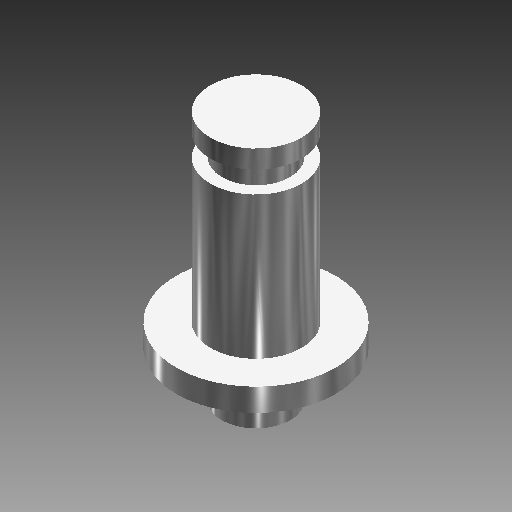
# Autodesk Inventor part: 308-16
Saved by Autodesk Inventor 2019 (Build 230136000, 136)
## iProperties
Company: Autodesk Inc.
Created: 2012-01-24
Part Number: 308-16
Material: Steel
Document SubType Name: Modeling
Designer: Autodesk Inc.
Mass: 1.16125 g
Surface Area: 2.26352 cm^2
Volume: 0.14793 cm^3
Density: 7.85 g/cm^3
Appearance: Chrome - Polished
Author: Inventor
Autodesk Inventor part; units mm, degrees
ref_plane "YZ Plane" through (0, 0, 0) normal (1, 0, 0) x (0, 1, 0)
ref_plane "XZ Plane" through (0, 0, 0) normal (0, 1, 0) x (-1, 0, 0)
ref_plane "XY Plane" through (0, 0, 0) normal (0, 0, 1) x (1, 0, 0)
sketch "Sketch1" plane through (0, 0, 0) normal (0, 0, 1) x (1, 0, 0)
  line L0 (0, 0) -> (1.5, 0)
  line L1 (1.5, 0) -> (1.5, 2)
  line L2 (1.5, 2) -> (0, 2)
  line L3 (0, 2) -> (0, 0)
  line L4 (0, 2) -> (3.5, 2)
  line L5 (3.5, 2) -> (3.5, 3)
  line L6 (3.5, 3) -> (0, 3)
  line L7 (0, 3) -> (0, 2)
  line L8 (0, 3) -> (2, 3)
  line L9 (2, 3) -> (2, 9.25)
  line L10 (2, 9.25) -> (0, 9.25)
  line L11 (0, 9.25) -> (0, 3)
  line L12 (0, 9.25) -> (1.5, 9.25)
  line L13 (1.5, 9.25) -> (1.5, 10.2)
  line L14 (1.5, 10.2) -> (0, 10.2)
  line L15 (0, 10.2) -> (0, 9.25)
  line L16 (0, 10.2) -> (2, 10.2)
  line L17 (2, 10.2) -> (2, 11)
  line L18 (2, 11) -> (0, 11)
  line L19 (0, 11) -> (0, 10.2)
  dimension "d8" = 4
  dimension "d9" = 3
  dimension "d10" = 8
  dimension "d11" = 9
  dimension "d12" = 11
  dimension "d13" = 0.8
  dimension "d14" = 1.75
  dimension "d16" = 7
  constraints: 40 end point, 11 parallel, 5 horizontal, 5 perpendicular, 1 collinear
  measures "d8" diameter of L17 L19
  measures "d9" diameter of L13 L19
  measures "d10" distance between parallel lines of L6 L18
  measures "d11" distance between parallel lines of L4 L18
  measures "d12" distance between parallel lines of L0 L18
  measures "d13" distance of L16.end L17.end
  measures "d14" distance between parallel lines of L10 L18
  measures "d16" diameter of L5 L3
revolve "Revolution1" add sketch "Sketch1" angle 360 about axis through (0, 9.25, 0) along (0, -1, 0)
body "Solid1"
